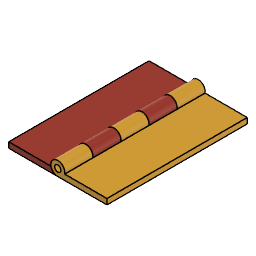
ex2 (Autodesk Fusion 360 design; units mm, degrees)
part number: 2026-03-30-19-41-59-000
part number: 2026-03-31-17-33-03-915
part number: 2026-03-31-17-33-06-995
Autodesk Fusion 360 part; units mm, degrees
sketch "Sketch3" plane through (0, 0, 0) normal (0, 1, 0) x (1, 0, 0)
  line L0 (0, 0) -> (35, 0)
  line L1 (35, 0) -> (35, -4)
  line L2 (35, -4) -> (4.899, -4)
  circle A0 centre (0, -5) radius 5
  circle A1 centre (0, -5) radius 2.2361
  line L3 (0, 0) -> (0, -5) construction
  dimension "d23" = 4
  dimension "d24" = 10
  dimension "d25" = 4.4721
  dimension "d26" = 35
  dimension "d27" = 5
  constraint horizontal L0
  constraint vertical L1
  constraint horizontal L2
  constraint coincident L0.start L3.start
  constraint concentric A0 A1
  constraint coincident A0 L2.end
  constraint coincident A0.centre A1.centre
  constraint perpendicular L0 L3
  measures "d23" distance of L0 L2
  measures "d24" diameter of A0
  measures "d25" diameter of A1
  measures "d26" distance of L1 A0.centre
  measures "d27" distance of L0 A0.centre
extrude "Extrude6" add sketch "Sketch3" along normal blind 100 makes body 1
extrude "Extrude7" add sketch "Sketch3" along normal blind 100 separate body makes body 2
extrude "Extrude8" cut sketch "Sketch3" along normal blind 20 from surface at 20 contours A0 bodies 2
extrude "Extrude9" cut sketch "Sketch3" along normal blind 20 from surface at 60 contours A0 bodies 2
move_body "Move5" bodies 1 to x (-1, 0, 0) y (0, -1, 0) z (0, 0, 1) at (-17.6966, 107.5097, 7.0748)
sketch "Sketch4" plane through (0, 7.5097, 0) normal (0, -1, 0) x (1, 0, 0)
  circle A0 centre (-17.6966, 12.0748) radius 2.2361
  line L0 (-52.6966, 7.0748) -> (-17.6966, 7.0748)
  arc A1 (-17.6966, 7.0748) -> (-22.5956, 11.0748) centre (-17.6966, 12.0748) ccw
  line L1 (-22.5956, 11.0748) -> (-52.6966, 11.0748)
  line L2 (-52.6966, 11.0748) -> (-52.6966, 7.0748)
  circle A2 centre (-17.6966, 12.0748) radius 2.2361
  circle A3 centre (-17.6966, 12.0748) radius 5
  constraint concentric A0 A2
  constraint concentric A2 A3
extrude "Extrude10" cut sketch "Sketch4" against normal blind 20 contours A1 A3 bodies 1
extrude "Extrude11" cut sketch "Sketch4" against normal blind 20 from surface at -40 contours A1 A3 bodies 1
extrude "Extrude12" cut sketch "Sketch4" against normal blind 20 from surface at -80 contours A1 A3 bodies 1
copy_body "Body->Comp1" bodies 1 removing the originals makes body 3 in component "stanga"
copy_body "Body->Comp2" bodies 2 removing the originals makes body 4 in component "dreapta"
move_body "Move1" bodies 3 to x (1, 0, 0) y (0, 1, 0) z (0, 0, 1) at (-3.0727, -2.4459, -7.0896) in component "stanga"
move_body "Move1'" bodies 4 to x (1, 0, 0) y (0, 1, 0) z (0, 0, 1) at (-3.0727, -2.4459, -7.0896) in component "dreapta"
component "stanga" placed x (1, 0, 0) y (0, 1, 0) z (0, 0, 1) at (0, 0, 0)
component "dreapta" placed x (1, 0, 0) y (0, 1, 0) z (0, 0, 1) at (-17.6966, 7.5097, 7.0748)
named bodies: "stanga", "dreapta"
